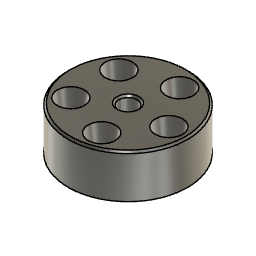
PCR_Heater v4 (Autodesk Fusion 360 design; units mm, degrees)
Autodesk Fusion 360 part; units mm, degrees
sketch "Sketch3" plane through (0, 0, 0) normal (0, 0, 1) x (1, 0, 0)
  circle A0 centre (0, 0) radius 9.75
  circle A1 centre (0, 0) radius 1.5
  dimension "d3" = 19.5
  dimension "d4" = 3
  constraint coincident A0.centre A1.centre
  measures "d3" diameter of A0
  measures "d4" diameter of A1
extrude "Extrude1" add sketch "Sketch3" along normal blind 7.1
sketch "Sketch6" plane through (0, 0, 7.1) normal (0, 0, 1) x (-1, 0, 0)
  circle A0 centre (0, 0) radius 1.5
  circle A1 centre (0, 0) radius 9.75
  circle A2 centre (-6.7, 0) radius 2.2159
  dimension "d15" = 4.4317
  dimension "d16" = 6.7
  measures "d15" diameter of A2
  measures "d16" distance of A0.centre A2.centre
extrude "Extrude4" cut sketch "Sketch6" against normal blind 5.3 draft -8.75 contours A2
sphere "SpherePrimitive1" cut diameter 2.8 placed x (-1, 0, 0) y (0, -1, 0) z (0, 0, 1) at (6.7, 0, 1.8)
pattern_circular "C-Pattern1" count 5 over 360 about axis through (0, 0, 7.1) along (0, 0, -1) of "Extrude4", "SpherePrimitive1"
chamfer "Chamfer1" distance 0.3 angle 45 1 edges at (-9.0902, -3.5258, 7.1)
chamfer "Chamfer2" distance 0.3 angle 45 1 edges at (-1.3985, 0.5424, 7.1)
extrude "Extrude2" [suppressed]
sketch "Sketch5" plane through (0, 0, 7.1) normal (0, 0, 1) x (-1, 0, 0)
  circle A0 centre (6.7, 0) radius 1.4
  circle A1 centre (0, 0) radius 1.5
  circle A2 centre (0, 0) radius 9.75
  circle A3 centre (6.7, 0) radius 2.215
  dimension "d12" = 4.43
  constraint concentric A0 A3
  measures "d12" diameter of A3
